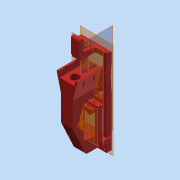
# Autodesk Inventor part: 08_Opentrons_Autofocus_flexurebaering
Saved by Autodesk Inventor 2019.4 (Build 234330000, 330)
## iProperties
Created: 2020-11-20
Part Number: 08_Opentrons_Autofocus_flexurebaering
Material: Generic
Document SubType Name: Modeling
Designer: diederichbenedict
Density: 1 g/cm^3
Appearance: Light Red
Author: diederichbenedict
Autodesk Inventor part; units mm, degrees
ref_plane "YZ Plane" through (0, 0, 0) normal (1, 0, 0) x (0, 1, 0)
ref_plane "XZ Plane" through (0, 0, 0) normal (0, 1, 0) x (-1, 0, 0)
ref_plane "XY Plane" through (0, 0, 0) normal (0, 0, 1) x (1, 0, 0)
ref_plane "Work Plane1" through (0, 0, 0) normal (0, 0, 1) x (1, 0, 0)
sketch "Sketch1" plane through (0, 0, 0) normal (0, 0, 1) x (1, 0, 0)
  line L0 (17.1585, 59.9787) -> (2.1585, 59.9787) construction
  line L1 (2.1585, 59.9787) -> (2.1585, 62.7008) construction
  line L2 (2.1585, 62.7008) -> (17.1585, 62.7008) construction
  line L3 (17.1585, 62.7008) -> (17.1585, 91.3397) construction
  line L4 (6.8647, 91.3397) -> (-18.8415, 91.3397) construction
  line L5 (-18.8415, 91.3397) -> (-18.8415, -14.6603) construction
  line L6 (-18.8415, -14.6603) -> (17.1585, -14.6603) construction
  line L7 (17.1585, -14.6603) -> (17.1585, 59.9787) construction
  line L8 (13.8585, 17.3397) -> (13.863, 4.6397) construction
  line L9 (13.863, 4.6397) -> (6.6783, 4.6397) construction
  arc A0 (-15.6915, 17.3397) -> (6.6783, 4.6397) centre (-0.9353, 17.2801) ccw construction
  arc A1 (6.6783, 30.0397) -> (-15.6915, 17.3397) centre (-0.9353, 17.3993) ccw construction
  line L10 (13.863, 30.0397) -> (6.6783, 30.0397) construction
  line L11 (13.8585, 17.3397) -> (13.863, 30.0397) construction
  circle A2 centre (-0.9353, 17.3993) radius 10.125 projected
  line L12 (17.1585, -14.6603) -> (-0.9353, -14.6603)
  line L13 (-0.9353, -14.6603) -> (-0.9353, -0.6603)
  line L14 (-0.9353, -0.6603) -> (17.1585, -0.6603)
  line L15 (17.1585, -0.6603) -> (17.1585, -14.6603)
  line L16 (17.1585, 0.8765) -> (13.1585, 0.8765)
  line L17 (13.1585, 0.8765) -> (13.1585, 91.3397)
  line L18 (13.1585, 91.3397) -> (17.1585, 91.3397)
  line L19 (13.1585, 34.2801) -> (-0.9353, 34.2801)
  line L20 (-0.9353, 34.2801) -> (-0.9353, 38.2801)
  line L21 (-0.9353, 38.2801) -> (13.1585, 38.2801)
  line L22 (13.1585, 38.2801) -> (13.1585, 34.2801)
  line L23 (13.1585, 91.3397) -> (-0.9353, 91.3397)
  line L24 (-0.9353, 91.3397) -> (-0.9353, 86.3397)
  line L25 (-0.9353, 86.3397) -> (13.1585, 86.3397)
  line L26 (13.1585, 86.3397) -> (13.1585, 91.3397)
  line L27 (-0.9353, 91.3397) -> (2.0647, 91.3397)
  line L28 (2.0647, 91.3397) -> (2.0647, 103.3397)
  line L29 (2.0647, 103.3397) -> (-0.9353, 103.3397)
  line L30 (-0.9353, 103.3397) -> (-0.9353, 91.3397)
  arc A3 (-5.6352, 28.9821) -> (3.1207, 29.223) centre (-0.9353, 17.3993) ccw projected
  arc A4 (-5.6352, 28.9821) -> (3.1207, 29.223) centre (-0.9353, 17.3993) ccw projected
  line L31 (14.1116, -3.6603) -> (2.1116, -3.6603) construction
  line L32 (2.1116, -3.6603) -> (2.1116, -11.6603) construction
  line L33 (2.1116, -11.6603) -> (14.1116, -11.6603) construction
  line L34 (14.1116, -11.6603) -> (14.1116, -3.6603) construction
  line L35 (14.1116, -3.6603) -> (2.1116, -11.6603) construction
  line L36 (2.1116, -3.6603) -> (14.1116, -11.6603) construction
  circle A5 centre (14.1116, -3.6603) radius 1.45
  circle A6 centre (14.1116, -11.6603) radius 1.45
  circle A7 centre (2.1116, -3.6603) radius 1.45
  circle A8 centre (2.1116, -11.6603) radius 1.45
  circle A9 centre (-0.9353, 17.3993) radius 10.125 projected
  circle A10 centre (7.7223, -11.6603) radius 1.45
  circle A11 centre (7.7223, -3.6603) radius 1.45
  circle A12 centre (-8.8475, 49.7489) radius 1.45 projected
  circle A13 centre (-9.593, -3.6603) radius 1.45 projected
  circle A14 centre (7.7223, -3.6603) radius 1.45 projected
  circle A15 centre (14.1116, -11.6603) radius 1.45 projected
  circle A16 centre (7.7223, -11.6603) radius 1.45 projected
  circle A17 centre (-9.593, -11.6603) radius 1.45 projected
  circle A18 centre (-15.9823, -11.6603) radius 1.45 projected
  circle A19 centre (6.9768, 49.7489) radius 1.45 projected
  line L37 (17.1585, 91.3397) -> (6.8647, 91.3397) projected
  arc A20 (17.1585, 76.0291) -> (17.1585, 46.2316) centre (138.7007, 61.1303) ccw
  line L38 (17.1585, 91.3397) -> (17.1585, 76.0291)
  line L39 (17.1585, 46.2316) -> (17.1585, 0.8765)
  point P0 (8.1116, -7.6603)
  dimension "d19" = 14
  dimension "d20" = 4
  dimension "d21" = 4
  dimension "d37" = 5
  dimension "d38" = 3
  dimension "d39" = 12
  dimension "d41" = 17
  dimension "d60" = 0
  dimension "d61" = 0
  dimension "d62" = 0
  dimension "d63" = 12
  dimension "d64" = 8
  dimension "d65" = 2.9
  dimension "d66" = 2.9
  dimension "d67" = 2.9
  dimension "d68" = 2.9
  dimension "d83" = 2.9
  dimension "d84" = 2.9
  constraints: 55 end point, 13 parallel, 7 centre point, 6 horizontal, 6 perpendicular, 6 point on line, 4 coincident, 2 midpoint, 2 point on circle
  measures "d19" distance of L12.end L13.end
  measures "d20" distance of L17.end L18.end
  measures "d21" distance of L19.end L20.end
  measures "d37" distance of L24.end L23.end
  measures "d38" distance of L29.end L28.end
  measures "d39" distance of L28.end L27.end
  measures "d41" distance from line of L19 A0.centre
  measures "d60" distance from line of L13 A0.centre
  measures "d61" distance from line of A0.centre L20
  measures "d62" distance from line of A1.centre L24
  measures "d63" distance of L33.end L32.end
  measures "d64" distance of L32.end L31.end
  measures "d65" diameter of A5
  measures "d66" diameter of A6
  measures "d67" diameter of A7
  measures "d68" diameter of A8
  measures "d83" diameter of A10
  measures "d84" diameter of A11
extrude "Extrusion1" add sketch "Sketch1" along normal blind 6 contours L12 L13 L14 L15 | L16 L17 L18 L38 A20 L39 | L19 L20 L21 L17 | L25 L24 L23 L17 | A5 | A7 | A8
ref_plane "Work Plane2" through (0, 0, 11) normal (0, 0, 1) x (1, 0, 0)
sketch "Sketch2" plane through (0, 0, 11) normal (0, 0, 1) x (1, 0, 0)
  line L0 (-0.9353, 34.2801) -> (13.1585, 34.2801) projected
  line L1 (13.1585, 34.2801) -> (13.1585, 0.8765) projected
  line L2 (13.1585, 0.8765) -> (17.1585, 0.8765) projected
  line L3 (17.1585, 76.0291) -> (17.1585, 91.3397) construction
  line L4 (17.1585, 91.3397) -> (-0.9353, 91.3397) construction
  line L5 (13.1585, 86.3397) -> (13.1585, 38.2801) construction
  line L6 (13.1585, 38.2801) -> (-0.9353, 38.2801) projected
  line L7 (-0.9353, 38.2801) -> (-0.9353, 34.2801) projected
  line L8 (13.1585, 38.2801) -> (-0.9353, 38.2801) projected
  line L9 (13.1585, 38.2801) -> (17.1585, 38.2801)
  line L10 (17.1585, 91.3397) -> (-0.9353, 91.3397) construction
  line L11 (13.1585, 91.3397) -> (-0.9353, 91.3397) construction
  line L12 (-0.9353, 91.3397) -> (-0.9353, 86.3397) construction
  line L13 (-0.9353, 86.3397) -> (13.1585, 86.3397) construction
  line L14 (13.1585, 86.3397) -> (13.1585, 91.3397) construction
  line L15 (-0.9353, 91.3397) -> (2.0647, 91.3397) construction
  line L16 (2.0647, 91.3397) -> (2.0647, 99.3397) construction
  line L17 (2.0647, 99.3397) -> (-0.9353, 99.3397) construction
  line L18 (-0.9353, 99.3397) -> (-0.9353, 91.3397) construction
  line L19 (-0.9353, 91.3397) -> (-0.9353, 86.3397) construction
  line L20 (-0.9353, 86.3397) -> (13.1585, 86.3397) construction
  line L21 (17.1585, 0.8765) -> (17.1585, 46.2316) projected
  arc A0 (17.1585, 76.0291) -> (17.1585, 46.2316) centre (138.7007, 61.1303) ccw construction
  line L22 (-0.9353, 38.2801) -> (13.1585, 38.2801) projected
  line L23 (-0.9353, 38.2801) -> (17.1585, 38.2801)
  line L24 (17.1585, 38.2801) -> (17.1585, 34.2801)
  line L25 (17.1585, 34.2801) -> (-0.9353, 34.2801)
  line L26 (-0.9353, 34.2801) -> (-0.9353, 38.2801)
  line L27 (13.1585, 0.8765) -> (17.1585, 0.8765) projected
  line L28 (17.1585, 34.2801) -> (13.1585, 34.2801)
  line L29 (13.1585, 34.2801) -> (13.1585, 0.8765)
  line L30 (13.1585, 0.8765) -> (17.1585, 0.8765)
  line L31 (17.1585, 0.8765) -> (17.1585, 34.2801)
  point P0 (0, 0)
  point P1 (2.0647, 91.3397)
  dimension "d34" = 5
  dimension "d35" = 3
  dimension "d36" = 8
  constraints: 34 end point, 8 parallel, 5 perpendicular, 4 horizontal, 2 point on line
  measures "d34" distance of L12.end L10.end
  measures "d35" distance of L17.end L16.end
  measures "d36" distance of L16.end L15.end
extrude "Extrusion2" add sketch "Sketch2" along normal blind 5
sketch "Sketch3" plane through (17.1585, -14.6603, 0) normal (1, 0, 0) x (0, 0, -1)
  line L0 (0, 14) -> (0, 0) projected
  line L1 (0, 14) -> (-6, 14) projected
  line L2 (-6, 0) -> (-6, 14) projected
  line L3 (0, 0) -> (-6, 0) projected
  line L4 (0, 90.6894) -> (0, 106) projected
  line L5 (0, 106) -> (-6, 106) projected
  line L6 (-6, 90.6894) -> (-6, 106) projected
  line L7 (-11, 106) -> (-11, 94.7976) projected
  line L8 (-16, 94.7976) -> (-16, 106) projected
  line L9 (-6, 14) -> (-6, 0) projected
  line L10 (-11.5, 14.0368) -> (-6, 14.0368)
  line L11 (-6, 14.0368) -> (-6, 9.0368)
  line L12 (-6, 9.0368) -> (-11.5, 9.0368)
  line L13 (-11.5, 9.0368) -> (-11.5, 14.0368)
  line L14 (-11, 15.5368) -> (-16, 15.5368) projected
  line L15 (-11, 15.5368) -> (-11.5, 15.5368)
  line L16 (-11.5, 15.5368) -> (-11.5, 14.0368)
  line L17 (-11.5, 14.0368) -> (-11, 14.0368)
  line L18 (-11, 14.0368) -> (-11, 15.5368)
  line L19 (0, 15.5368) -> (-0.5, 15.5368)
  line L20 (-0.5, 15.5368) -> (-0.5, 14)
  line L21 (-0.5, 14) -> (0, 14)
  line L22 (0, 14) -> (0, 15.5368)
  line L23 (-6, 15.5368) -> (-6, 106) projected
  line L24 (-6, 54.4404) -> (-11.5, 54.4404)
  line L25 (-11.5, 54.4404) -> (-11.5, 59.4404)
  line L26 (-11.5, 59.4404) -> (-6, 59.4404)
  line L27 (-6, 59.4404) -> (-6, 54.4404)
  line L28 (-11, 52.9404) -> (-16, 52.9404) projected
  line L29 (-11, 52.9404) -> (-11.5, 52.9404)
  line L30 (-11.5, 52.9404) -> (-11.5, 54.4404)
  line L31 (-11.5, 54.4404) -> (-11, 54.4404)
  line L32 (-11, 54.4404) -> (-11, 52.9404)
  line L33 (0, 90.6894) -> (-6, 90.6894) projected
  line L34 (-11, 106) -> (-16, 106) projected
  line L35 (-11, 94.7976) -> (-16, 94.7976) projected
  point P0 (0, 14.6603)
  dimension "d25" = 5
  dimension "d26" = 0.5
  dimension "d27" = 0.5
  dimension "d28" = 5
  dimension "d29" = 0.5
  dimension "d40" = 0
  constraints: 40 end point, 10 parallel, 6 point on line, 5 horizontal, 5 perpendicular
  measures "d25" distance of L10.end L11.end
  measures "d26" distance of L17.end L16.end
  measures "d27" distance of L21.end L20.end
  measures "d28" distance of L24.end L25.end
  measures "d29" distance of L30.end L31.end
  measures "d40" distance between parallel lines of L30 L25
extrude "Extrusion3" add sketch "Sketch3" against normal up to surface (4 mm away) contours L1 L20 L19 L22 | L2 L12 L13 L10 L11 | L10 L16 L14 L18
ref_plane "Work Plane3" through (0, 0, 18) normal (0, 0, 1) x (1, 0, 0)
sketch "Sketch4" plane through (0, 0, 18) normal (0, 0, 1) x (1, 0, 0)
  line L0 (17.1585, 34.8891) -> (-18.8415, 34.8891)
  line L1 (-0.9353, 34.2801) -> (13.1585, 34.2801) projected
  line L2 (13.1585, 34.2801) -> (13.1585, 0.8765) projected
  line L3 (13.1585, 0.8765) -> (17.1585, 0.8765) projected
  line L4 (-0.9353, 38.2801) -> (-0.9353, 34.2801) projected
  line L5 (-4.5265, 27.3641) -> (2.6559, 27.3641) projected
  arc A0 (9.49, 15.527) -> (2.6559, 27.3641) centre (-0.9353, 17.3993) ccw projected
  line L6 (9.49, 15.527) -> (5.8988, 9.3069) projected
  arc A1 (-7.7695, 9.3069) -> (5.8988, 9.3069) centre (-0.9353, 17.3993) ccw projected
  line L7 (-7.7695, 9.3069) -> (-11.3607, 15.527) projected
  arc A2 (-4.5265, 27.3641) -> (-11.3607, 15.527) centre (-0.9353, 17.3993) ccw projected
  arc A3 (-3.2146, 30.3993) -> (-4.8009, 29.6174) centre (-3.2146, 28.3993) ccw projected
  arc A4 (-5.6352, 28.9821) -> (-4.8009, 29.6174) centre (-6.3872, 30.8354) ccw projected
  arc A5 (-5.6352, 28.9821) -> (3.1207, 29.223) centre (-0.9353, 17.3993) ccw projected
  arc A6 (2.3012, 29.7571) -> (3.1207, 29.223) centre (3.7697, 31.1148) ccw projected
  arc A7 (2.3012, 29.7571) -> (0.8326, 30.3993) centre (0.8326, 28.3993) ccw projected
  line L8 (0.8326, 30.3993) -> (-3.2146, 30.3993) projected
  arc A8 (2.4113, 29.8589) -> (0.8326, 30.5493) centre (0.8326, 28.3993) ccw
  arc A9 (2.4113, 29.8589) -> (3.1694, 29.3649) centre (3.7697, 31.1148) ccw
  arc A10 (-5.6916, 29.1211) -> (3.1694, 29.3649) centre (-0.9353, 17.3993) ccw
  arc A11 (-5.6916, 29.1211) -> (-4.9199, 29.7087) centre (-6.3872, 30.8354) ccw
  arc A12 (-3.2146, 30.5493) -> (-4.9199, 29.7087) centre (-3.2146, 28.3993) ccw
  line L9 (-3.2146, 30.5493) -> (0.8326, 30.5493)
  line L10 (8.265, 26.0813) -> (11.869, 29.6852)
  line L11 (8.265, 26.0813) -> (13.3617, 26.0813) construction
  line L12 (11.869, 29.6852) -> (11.869, 32.7801)
  line L13 (11.869, 32.7801) -> (-0.9353, 32.7801)
  line L14 (-0.9353, 38.2801) -> (-0.9353, 34.2801) projected
  line L15 (-0.9353, 33.5573) -> (-0.9353, 30.5493)
  line L16 (-0.9353, 32.7801) -> (-0.9353, 30.5493)
  line L17 (17.1585, 0.8765) -> (17.1585, 38.2801) construction
  line L18 (17.1585, 0.8765) -> (17.1585, 38.2801) projected
  line L19 (17.1585, 0.8765) -> (17.1585, 34.8891)
  line L20 (17.1585, 38.2801) -> (-0.9353, 38.2801) projected
  point P0 (0, 0)
  point P1 (17.1585, 49.7489)
  dimension "d43" = 0.15
  dimension "d44" = 45
  dimension "d49" = 1.5
  constraints: 18 end point, 11 point on circle, 5 centre point, 4 point on line, 2 horizontal, 2 vertical, 1 collinear, 1 equal length, 1 perpendicular, 7 other
  measures "d43" radial gap between concentric circles of A7 A8
  measures "d44" angle of L11 L10
  measures "d49" distance between parallel lines of L1 L13
extrude "Extrusion4" add sketch "Sketch4" against normal up to surface (18 mm away) contours A8 L9 L15 L13 L12 L10 A10 A9
sketch "Sketch5" plane through (-0.9353, 30.5493, 18) normal (-1, 0, 0) x (0, 0, 1)
  line L0 (-7, 3.7307) -> (-7, 7.7307) projected
  line L1 (-7, 3.7307) -> (-2, 3.7307) projected
  line L2 (-2, 7.7307) -> (-2, 3.7307) projected
  line L3 (-7, 7.7307) -> (-2, 7.7307) projected
  line L4 (-18, 0) -> (-18, 2.2307) projected
  line L5 (0, 0) -> (-18, 0) projected
  line L6 (0, 2.2307) -> (0, 0) projected
  line L7 (0, 2.2307) -> (-18, 2.2307) projected
  line L8 (-18, 3.7307) -> (-18, 7.7307) projected
  line L9 (-18, 3.7307) -> (-12, 3.7307) projected
  line L10 (-12, 7.7307) -> (-12, 3.7307) projected
  line L11 (-18, 7.7307) -> (-12, 7.7307) projected
  line L12 (0, 2.2307) -> (-18, 2.2307) projected
  line L13 (-18, 3.7307) -> (-17.5, 3.7307)
  line L14 (-17.5, 3.7307) -> (-17.5, 2.2307)
  line L15 (-17.5, 2.2307) -> (-18, 2.2307)
  line L16 (-18, 2.2307) -> (-18, 3.7307)
  line L17 (-7, 3.7307) -> (-6.5, 3.7307)
  line L18 (-6.5, 3.7307) -> (-6.5, 2.2307)
  line L19 (-6.5, 2.2307) -> (-7, 2.2307)
  line L20 (-7, 2.2307) -> (-7, 3.7307)
  point P0 (-18, -30.5493)
  dimension "d47" = 0.5
  dimension "d48" = 0.5
  constraints: 16 end point, 4 parallel, 2 horizontal, 2 perpendicular, 2 point on line
  measures "d47" distance of L14.end L15.end
  measures "d48" distance of L18.end L19.end
sketch "Sketch7" plane through (-0.9353, 32.7801, 18) normal (0, 1, 0) x (1, 0, 0)
  circle A0 centre (-0.2556, 2.7408) radius 1.45 projected
  line L0 (-0.2556, 2.7408) -> (-0.2556, 18) construction
  line L1 (1.3944, 2.7408) -> (1.3944, 18)
  line L2 (-1.9056, 18) -> (-1.9056, 2.7408)
  arc A1 (-1.9056, 2.7408) -> (1.3944, 2.7408) centre (-0.2556, 2.7408) ccw
  arc A2 (1.3944, 18) -> (-1.9056, 18) centre (-0.2556, 18) ccw
  line L3 (-0.2556, 2.7408) -> (15.0036, 2.7408) construction
  point P0 (0.9353, 18)
  point P1 (-0.2556, 10.3704)
  dimension "d50" = 90
  dimension "d51" = 0.2
  constraints: 10 end point, 4 point on circle, 4 tangent, 2 centre point, 1 horizontal, 1 midpoint, 1 parallel, 1 perpendicular
  measures "d50" angle of L3 L0
  measures "d51" radial gap between concentric circles of A0 A1
extrude "Extrusion5" cut sketch "Sketch7" against normal blind 5 contours A0 | A1 L2 A2 L1
extrude "Extrusion6" add sketch "Sketch5" against normal up to surface (12.8043 mm away) contours L1 L18 L7 L20 | L7 L16 L9 L14
sketch "Sketch8" plane through (0, 0, 18) normal (0, 0, 1) x (1, 0, 0)
  arc A0 (2.4113, 29.8589) -> (0.8326, 30.5493) centre (0.8326, 28.3993) ccw projected
  arc A1 (2.4113, 29.8589) -> (3.1694, 29.3649) centre (3.7697, 31.1148) ccw projected
  arc A2 (8.265, 26.0813) -> (3.1694, 29.3649) centre (-0.9353, 17.3993) ccw projected
  line L0 (8.265, 26.0813) -> (11.869, 29.6852) projected
  line L1 (11.869, 29.6852) -> (11.869, 32.7801) projected
  line L2 (11.869, 32.7801) -> (-0.9353, 32.7801) projected
  line L3 (-0.9353, 32.7801) -> (-0.9353, 30.5493) projected
  line L4 (-0.9353, 30.5493) -> (0.8326, 30.5493) projected
  line L5 (11.869, 34.2801) -> (11.869, 32.7801) projected
  line L6 (-0.9353, 34.2801) -> (11.869, 34.2801) projected
  line L7 (-0.9353, 32.7801) -> (-0.9353, 34.2801) projected
  line L8 (-0.9353, 32.7801) -> (0.459, 32.7801) projected
  line L9 (11.869, 32.7801) -> (0.459, 32.7801) projected
  line L10 (-0.8954, 34.2801) -> (2.6046, 34.2801)
  line L11 (2.6046, 34.2801) -> (2.6046, 31.7801)
  line L12 (2.6046, 31.7801) -> (-0.8954, 31.7801)
  line L13 (-0.8954, 31.7801) -> (-0.8954, 34.2801)
  point P0 (0, 0)
  dimension "d56" = 3.5
  dimension "d57" = 2.5
  constraints: 8 end point, 2 parallel, 1 horizontal, 1 perpendicular, 1 point on line
  measures "d56" distance of L11.end L12.end
  measures "d57" distance of L10.end L11.end
extrude "Extrusion7" cut sketch "Sketch8" against normal through all contours L13 L6 L11 L2 | L2 L11 L12 L13
sketch "Sketch9" plane through (-0.9353, -14.6603, 0) normal (-1, 0, 0) x (0, 0, 1)
  line L0 (0, 0) -> (0, 14) projected
  line L1 (0, 0) -> (6, 0) projected
  line L2 (6, 14) -> (6, 0) projected
  line L3 (0, 14) -> (6, 14) projected
  line L4 (24.0519, 27.1099) -> (31.123, 34.181) projected
  line L5 (29.7087, 35.5952) -> (22.6377, 28.5241) projected
  line L6 (31.123, 34.181) -> (29.7087, 35.5952)
  line L7 (24.0519, 27.1099) -> (22.6377, 28.5241)
  line L8 (29.7087, 35.7366) -> (22.4963, 28.5241)
  line L9 (24.0519, 26.9685) -> (31.2644, 34.181)
  line L10 (31.2644, 34.181) -> (29.7087, 35.7366)
  line L11 (22.4963, 28.5241) -> (38.5218, 28.5241) construction
  line L12 (0, 14) -> (6, 14) projected
  line L13 (15.7236, 14) -> (6, 14)
  line L14 (6, 14) -> (6, 0)
  line L15 (29.7087, 35.7366) -> (29.7087, 57.7366)
  line L16 (29.7087, 57.7366) -> (0, 57.7366)
  line L17 (0, 101) -> (0, 52.9404) projected
  line L18 (0, 57.7366) -> (0, 63.7366)
  line L19 (0, 63.7366) -> (35.7087, 63.7366)
  line L20 (35.7087, 63.7366) -> (35.7087, 34.181)
  line L21 (35.7087, 34.181) -> (19.7699, 0)
  line L22 (0, 0) -> (6, 0) projected
  line L23 (19.7699, 0) -> (6, 0)
  line L24 (0, 57.7366) -> (22.1164, 54.292)
  line L25 (22.1164, 54.292) -> (29.7087, 35.7366)
  line L26 (15.7236, 14) -> (22.4963, 16.4302)
  line L27 (22.4963, 16.4302) -> (22.4963, 25.4128)
  line L28 (22.4963, 28.5241) -> (22.3727, 28.2591)
  line L29 (19.9014, 22.9594) -> (19.7778, 22.6944)
  line L30 (24.0519, 26.9685) -> (22.4963, 25.4128)
  line L31 (22.4963, 28.5241) -> (22.567, 28.4534)
  line L32 (23.9812, 27.0392) -> (24.0519, 26.9685)
  point P0 (0, 14.6603)
  dimension "d69" = 0.1
  dimension "d71" = 22
  dimension "d72" = 6
  dimension "d73" = 6
  constraints: 48 end point, 7 point on line, 4 perpendicular, 3 parallel, 2 vertical, 1 collinear, 1 horizontal, 3 other
  measures "d69" distance between parallel lines of L6 L10
  measures "d71" distance of L8.start L15.end
  measures "d72" distance of L16.end L18.end
  measures "d73" distance between parallel lines of L20 L15
extrude "Extrusion8" add sketch "Sketch9" against normal blind 7 contours L2 L13 L26 L27 L30 L9 L10 L15 L16 L17 L19 L20 L21 L23 | L16 L15 L25 L24
sketch "Sketch10" plane through (-0.9353, 19.5207, 35.7087) normal (0, 0, 1) x (1, 0, 0)
  line L0 (12.5, 51.9844) -> (-12.5, 51.9844) projected
  line L1 (0, 29.5556) -> (7, 29.5556) projected
  line L2 (12.5, 51.9844) -> (7, 29.5556)
  line L3 (0, 29.5556) -> (7, 29.5556) projected
  line L4 (0, 29.5556) -> (0, 46.1634)
  line L5 (0, 46.1634) -> (8.8956, 46.1634)
  line L6 (8.8956, 46.1634) -> (10.323, 51.9844)
  line L7 (12.5, 51.9844) -> (10.323, 51.9844)
  point P0 (0.9353, -19.5207)
  constraints: 10 end point, 2 parallel, 1 perpendicular, 1 point on line, 1 vertical
extrude "Extrusion9" add sketch "Sketch10" against normal up to surface (35.7087 mm away)
sketch "Sketch11" plane through (9.3877, 71.5051, 35.7087) normal (0, 1, 0) x (1, 0, 0)
  circle A0 centre (0.177, 22.0355) radius 1.05 projected
  circle A1 centre (0.177, 9.5355) radius 1.05 projected
  ellipse E0 centre (-10.323, 9.5355) end of major axis (-12.2552, 9.5355) minor radius 1.3663 projected
  circle A2 centre (-10.323, 9.5355) radius 5
  circle A3 centre (0.177, 22.0355) radius 0.95
  circle A4 centre (0.177, 9.5355) radius 0.95
  line L0 (-10.323, 18.8634) -> (-10.323, 34.9295) construction
  line L1 (-8.873, 20.3134) -> (-8.873, 33.4795)
  line L2 (-11.773, 33.4795) -> (-11.773, 20.3134)
  arc A5 (-11.773, 20.3134) -> (-8.873, 20.3134) centre (-10.323, 20.3134) ccw
  arc A6 (-8.873, 33.4795) -> (-11.773, 33.4795) centre (-10.323, 33.4795) ccw
  arc A7 (-10.2831, 18.8262) -> (-8.9287, 20.4495) centre (-10.5787, 20.4495) ccw projected
  point P0 (-9.3877, 35.7087)
  point P1 (-10.323, 26.8965)
  point P2 (-10.323, 35.2087)
  dimension "d78" = 10
  dimension "d79" = 1.9
  dimension "d80" = 1.9
  dimension "d99" = 2.9
  constraints: 8 end point, 6 point on circle, 5 centre point, 4 tangent, 3 coincident, 2 point on line, 1 midpoint, 1 parallel, 1 vertical, 1 other
  measures "d78" diameter of A2
  measures "d79" diameter of A3
  measures "d80" diameter of A4
  measures "d99" diameter of A6
extrude "Extrusion10" cut sketch "Sketch11" against normal up to surface (33.225 mm away) contours E0 | A2 | A3 | A4 | A5 L2 A6 L1
sketch "Sketch12" plane through (0, 0, 6) normal (0, 0, 1) x (1, 0, 0)
  line L0 (-0.9353, 19.5207) -> (-0.9353, 65.6841) projected
  line L1 (-0.9353, 19.5207) -> (6.0647, 19.5207) projected
  line L2 (6.0647, 49.0763) -> (6.0647, 19.5207) projected
  line L3 (6.0647, 49.0763) -> (11.5647, 71.5051) projected
  line L4 (11.5647, 71.5051) -> (9.3877, 71.5051) projected
  line L5 (9.3877, 71.5051) -> (7.9603, 65.6841) projected
  line L6 (7.9603, 65.6841) -> (-0.9353, 65.6841) projected
  line L7 (6.0647, 43.0763) -> (6.0647, 49.0763) projected
  line L8 (6.0647, 46.0763) -> (11.0647, 46.0763)
  line L9 (11.0647, 46.0763) -> (11.0647, 69.4661)
  circle A0 centre (6.9768, 49.7489) radius 1.45
  point P0 (0, 0)
  dimension "d85" = 5
  dimension "d86" = 2.9
  constraints: 4 end point, 1 centre point, 1 horizontal, 1 midpoint, 1 perpendicular, 1 point on line
  measures "d85" distance of L8.start L8.end
  measures "d86" diameter of A0
extrude "Extrusion11" add sketch "Sketch12" against normal up to surface (6 mm away) contours L2 A0 L3 L9 L8
mirror "Mirror2" about plane through (-0.9353, -0.6603, 0) normal (-1, 0, 0) of "Extrusion1", "Extrusion2", "Extrusion3", "Extrusion4", "Extrusion5", "Extrusion6", "Extrusion7", "Extrusion8", "Extrusion9", "Extrusion10", "Extrusion11"
fillet "Fillet1" radius 3 6 edges at (-19.0292, 91.3397, 3) (17.1585, 91.3397, 3) (13.1585, 86.3397, 3) (-15.0292, 86.3397, 3) (-0.9353, 19.5207, 35.7087) (-0.9353, -14.6603, 19.7699)
ref_plane "Work Plane8" through (-0.9353, 66.6068, 11.0279) normal (-1, 0, 0) x (0, 1, 0)
sketch "Sketch13" plane through (-0.9353, 66.6068, 11.0279) normal (-1, 0, 0) x (0, 1, 0)
  line L0 (24.7329, 5.0279) -> (24.7329, 11.0279) projected
  line L1 (19.7329, 5.0279) -> (24.7329, 5.0279)
  line L2 (24.7329, 5.0279) -> (24.7329, -14.9721)
  line L3 (24.7329, -14.9721) -> (19.7329, -14.9721)
  line L4 (19.7329, -14.9721) -> (19.7329, 5.0279)
  line L5 (24.7329, -14.9721) -> (39.7329, -14.9721)
  line L6 (39.7329, -14.9721) -> (39.7329, -9.9721)
  line L7 (39.7329, -9.9721) -> (24.7329, -9.9721)
  line L8 (24.7329, -9.9721) -> (24.7329, -14.9721)
  point P0 (-66.6068, 11.0279)
  dimension "d90" = 20
  dimension "d91" = 15
  dimension "d92" = 5
  constraints: 16 end point, 4 parallel, 2 horizontal, 2 perpendicular
  measures "d90" distance of L1.end L2.end
  measures "d91" distance of L7.end L6.end
  measures "d92" distance of L6.end L5.end
extrude "Extrusion12" add sketch "Sketch13" along normal mid plane 10
fillet "Fillet2" radius 2 6 edges at (-0.9353, 86.3397, 26) (-0.9353, 106.3397, 26) (-0.9353, 106.3397, 21) (-0.9353, 91.3397, 21) (-5.9353, 88.8397, 6) (4.0647, 88.8397, 6)
sketch "Sketch14" plane through (4.0647, 93.3397, 21) normal (0, 0, -1) x (-1, 0, 0)
  circle A0 centre (5, 7) radius 1.425 projected
  point P0 (4.0647, -93.3397)
extrude "Extrusion13" cut sketch "Sketch14" against normal blind 1
fillet "Fillet3" radius 2 2 edges at (0.4897, 100.3397, 21) (0.4897, 100.3397, 22)
sketch "Sketch15" plane through (-16.0292, 91.3397, 0) normal (0, 1, 0) x (1, 0, 0)
  arc A0 (13.6439, -15.3953) -> (16.5439, -15.3953) centre (15.0939, -15.3953) ccw projected
  line L0 (15.0939, -15.3953) -> (15.0939, -9.2086) construction
  line L1 (13.6439, -15.3953) -> (13.6439, -9.2086)
  line L2 (16.5439, -9.2086) -> (16.5439, -15.3953)
  arc A1 (13.6439, -15.3953) -> (16.5439, -15.3953) centre (15.0939, -15.3953) ccw
  arc A2 (16.5439, -9.2086) -> (13.6439, -9.2086) centre (15.0939, -9.2086) ccw
  point P0 (16.0292, 0)
  point P1 (15.0939, -12.302)
  constraints: 8 end point, 4 point on circle, 4 tangent, 2 centre point, 1 concentric, 1 midpoint, 1 parallel, 1 vertical
extrude "Extrusion14" cut sketch "Sketch15" against normal blind 10
sketch "Sketch16" plane through (17.1585, 76.0291, 6) normal (1, 0, 0) x (0, 0, -1)
  line L0 (0, 12.3106) -> (6, 12.3106) projected
  line L1 (0, 0) -> (0, 12.3106) projected
  line L2 (6, 0) -> (0, 0) projected
  line L3 (6, 0) -> (6, 12.3106) projected
  line L4 (-2, 15.3106) -> (-2, 10.3106) projected
  line L5 (-2, 15.3106) -> (-13, 15.3106) projected
  arc A0 (-15, 17.3106) -> (-13, 15.3106) centre (-13, 17.3106) ccw projected
  line L6 (-15, 17.3106) -> (-15, 28.3106) projected
  arc A1 (-15, 28.3106) -> (-17, 30.3106) centre (-17, 28.3106) ccw projected
  line L7 (-17, 30.3106) -> (-18, 30.3106) projected
  arc A2 (-18, 30.3106) -> (-20, 28.3106) centre (-18, 28.3106) ccw projected
  line L8 (-20, 28.3106) -> (-20, 12.3106) projected
  arc A3 (-20, 12.3106) -> (-18, 10.3106) centre (-18, 12.3106) ccw projected
  line L9 (-18, 10.3106) -> (-2, 10.3106) projected
  line L10 (6, 0) -> (6, 12.3106) projected
  line L11 (6, 12.3106) -> (-13, 15.3106)
  line L12 (-13, 15.3106) -> (-13, 18.1767)
  line L13 (-13, 18.1767) -> (10.2098, 18.781)
  line L14 (10.2098, 18.781) -> (6, 12.3106)
  point P0 (6, -76.0291)
  constraints: 8 end point, 1 point on circle, 1 vertical
extrude "Extrusion15" cut sketch "Sketch16" against normal through all contours L11 L4 L5 L12 L13 L14 | L11 L5 L4
sketch "Sketch17" plane through (-12.0292, 86.3397, 0) normal (0, -1, 0) x (1, 0, 0)
  arc A0 (9.6439, 9.2086) -> (12.5439, 9.2086) centre (11.0939, 9.2086) ccw projected
  line L0 (12.5439, 15.3953) -> (12.5439, 9.2086) projected
  arc A1 (12.5439, 15.3953) -> (9.6439, 15.3953) centre (11.0939, 15.3953) ccw projected
  line L1 (9.6439, 9.2086) -> (9.6439, 15.3953) projected
  ellipse E0 centre (26.1878, 0) end of major axis (26.1878, 19) minor radius 3 (29.1878, 0) -> (29.0343, 6) ccw projected
  line L2 (-7, 0) -> (29.1878, 0) projected
  ellipse E1 centre (-4, 0) end of major axis (-4, 19) minor radius 3 (-6.8465, 6) -> (-7, 0) ccw projected
  line L3 (4.0939, 6) -> (-6.8465, 6) projected
  arc A2 (4.0939, 6) -> (6.0939, 8) centre (4.0939, 8) ccw projected
  line L4 (6.0939, 19) -> (6.0939, 8) projected
  line L5 (16.0939, 19) -> (6.0939, 19) projected
  line L6 (16.0939, 8) -> (16.0939, 19) projected
  arc A3 (16.0939, 8) -> (18.0939, 6) centre (18.0939, 8) ccw projected
  line L7 (29.0343, 6) -> (18.0939, 6) projected
  line L8 (6.0939, 19) -> (16.0939, 19)
  line L9 (16.0939, 19) -> (16.0939, 24.7189)
  line L10 (16.0939, 24.7189) -> (6.0939, 24.7189)
  line L11 (6.0939, 24.7189) -> (6.0939, 19)
  line L12 (31.1878, -0.1624) -> (-9, -0.1624)
  line L13 (-9, -0.1624) -> (-9, 6)
  line L14 (-9, 6) -> (31.1878, 6)
  line L15 (31.1878, 6) -> (31.1878, -0.1624)
  line L16 (31.1878, -0.1624) -> (-9, 6) construction
  line L17 (-9, -0.1624) -> (31.1878, 6) construction
  line L18 (-7, 0) -> (-7, 6) projected
  line L19 (29.1878, 6) -> (29.1878, 0) projected
  point P0 (12.0292, 0)
  point P1 (11.0939, 2.9188)
  dimension "d104" = 2
  dimension "d105" = 2
  constraints: 20 end point, 4 parallel, 2 horizontal, 2 midpoint, 2 perpendicular, 2 other
  measures "d104" distance between parallel lines of L13 L18
  measures "d105" distance between parallel lines of L15 L19
extrude "Extrusion16" add sketch "Sketch17" along normal blind 2 contours L2 E1 L3 L14 L7 E0 | E0 L14 L19 | L18 L14 E1 | L14 A2 L4 L5 L6 A3 | L5 L11 L10 L9
sketch "Sketch18" plane through (7.9603, 65.6841, 35.7087) normal (0, 1, 0) x (1, 0, 0)
  circle A0 centre (-8.8956, 9.5355) radius 5 projected
  point P0 (-7.9603, 35.7087)
extrude "Extrusion17" cut sketch "Sketch18" against normal up to surface (46.1634 mm away)
ref_plane "Work Plane6" through (-1.8707, 0, 11) normal (0, 0, -1) x (-1, 0, 0)
ref_plane "Work Plane7" through (-1.8707, 0, 18) normal (0, 0, -1) x (-1, 0, 0)
body "Solid1"
